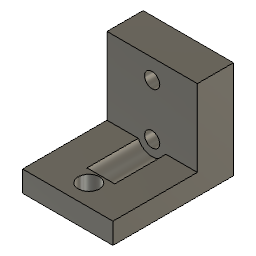
VerbindungMotorisierteLinearfuehrungQuerprofil (Autodesk Fusion 360 design; units mm, degrees)
part number: 2025-11-29-22-10-42-510
Autodesk Fusion 360 part; units mm, degrees
sketch "Skizze1" plane through (0, 0, 0) normal (0, 0, 1) x (1, 0, 0)
  line L0 (0, 0) -> (30, 0)
  line L1 (30, 0) -> (30, 40)
  line L2 (30, 40) -> (0, 40)
  line L3 (0, 40) -> (0, 0)
  dimension "d1" = 30
  dimension "d2" = 40
  constraint horizontal L0
  constraint vertical L1
  constraint horizontal L2
  constraint vertical L3
  constraint coincident L0.start L3.end
  measures "d1" distance of L0.start L0.end
  measures "d2" distance of L0.start L2.end
extrude "Extrusion1" add sketch "Skizze1" along normal blind 7 makes body 1
sketch "Skizze2" plane through (0, 0, 7) normal (0, 0, 1) x (-1, 0, 0)
  line L0 (0, -40) -> (0, 0)
  line L1 (0, 0) -> (-30, 0)
  line L2 (-30, 0) -> (-30, -40)
  line L3 (-30, -40) -> (0, -40)
  line L4 (0, -40) -> (-30, -40)
  line L5 (-30, -40) -> (-30, -28)
  line L6 (-30, -28) -> (0, -28)
  line L7 (0, -28) -> (0, -40)
  constraint horizontal L4
  constraint vertical L5
  constraint horizontal L6
  constraint vertical L7
  constraint coincident L2 L5.end
  constraint coincident L0.start L3.end
extrude "Extrusion2" add sketch "Skizze2" along normal blind 29 contours L0 L2 L3 L4 L5 L6 L7 bodies 1
sketch "Skizze3" plane through (0, 40, 0) normal (0, 1, 0) x (-1, 0, 0)
  line L0 (-30, 0) -> (0, 0)
  line L1 (0, 0) -> (0, 36)
  line L2 (0, 36) -> (-30, 36)
  line L3 (-30, 36) -> (-30, 0)
  line L4 (-15, 0) -> (-15, 36)
  line L5 (-15, 0) -> (-15, 13.5)
  circle A0 centre (-15, 13.5) radius 2.5
  line L6 (-15, 13.5) -> (-15, 30.5)
  circle A1 centre (-15, 30.5) radius 2.5
  dimension "d7" = 13.5
  dimension "d8" = 5
  dimension "d9" = 17
  dimension "d10" = 5
  constraint midpoint L0 L4.start
  constraint midpoint L2 L4.end
  constraint perpendicular L0 L5
  constraint coincident L5.end A0.centre
  constraint parallel L4 L6
  constraint coincident L6.end A1.centre
  measures "d7" distance of L4.start L5.end
  measures "d8" diameter of A0
  measures "d9" distance of L5.end L6.end
  measures "d10" diameter of A1
extrude "Extrusion3" add 1 faces at (20, 32, 36) along direction (0, 0, 1) blind 1 on bodies 1 bodies 1
extrude "Extrusion4" cut sketch "Skizze3" against normal blind 18 contours L4 L5 A0 L6 | L4 L5 A0 L6 | L4 L6 A1 | L4 L6 A1 bodies 1
sketch "Skizze4" plane through (0, 0, 7) normal (0, 0, 1) x (-1, 0, 0)
  line L0 (-30, -28) -> (0, -28)
  line L1 (0, -28) -> (0, 0)
  line L2 (0, 0) -> (-30, 0)
  line L3 (-30, 0) -> (-30, -28)
  line L4 (-15, -28) -> (-15, 0)
  line L5 (-15, 0) -> (-15, -7)
  circle A0 centre (-15, -7) radius 3.5
  line L6 (-15, -7) -> (-15, -21)
  circle A1 centre (-15, -21) radius 3.5
  dimension "d15" = 7
  dimension "d16" = 7
  dimension "d17" = 14
  dimension "d18" = 7
  constraint midpoint L0 L4.start
  constraint midpoint L2 L4.end
  constraint parallel L4 L5
  constraint coincident L5.end A0.centre
  constraint parallel L4 L6
  constraint coincident L6.end A1.centre
  measures "d15" distance of L4.end L5.end
  measures "d16" diameter of A0
  measures "d17" distance of L5.end L6.end
  measures "d18" diameter of A1
extrude "Extrusion5" cut sketch "Skizze4" against normal blind 7 contours L4 L5 A0 L6 | L4 L5 A0 L6 bodies 1
split "Teilen1" by plane through (0, 0, 7) normal (0, 0, 1) bodies 1 makes body 2 at (25.7508, 28, 24.4718)
move_body "Verschieben1" bodies 2 to x (1, 0, 0) y (0, 1, 0) z (0, 0, 1) at (0, 0, -4.5)
sketch "Skizze5" plane through (0, 0, 7) normal (0, 0, 1) x (-1, 0, 0)
  circle A0 centre (-15, -7) radius 3.5
  line L0 (0, -40) -> (0, 0)
  line L1 (0, 0) -> (-30, 0)
  line L2 (-30, 0) -> (-30, -40)
  line L3 (-30, -40) -> (0, -40)
  line L4 (0, -28) -> (-30, -28)
  line L5 (-15, -28) -> (-15, -14)
  constraint coincident L0 L4.start
  constraint coincident L2 L4.end
  constraint perpendicular L2 L4
  constraint midpoint L4 L5.start
  constraint perpendicular L4 L5
sketch "Skizze6" plane through (0, 28, 0) normal (0, -1, 0) x (1, 0, 0)
  circle A0 centre (15, 26) radius 2.5
  circle A1 centre (15, 9) radius 2.5
  line L0 (0, 2.5) -> (30, 2.5)
  line L1 (30, 2.5) -> (30, 32.5)
  line L2 (30, 32.5) -> (0, 32.5)
  line L3 (0, 32.5) -> (0, 2.5)
  circle A2 centre (15, 9) radius 2.5
  circle A3 centre (15, 9) radius 5
  dimension "d23" = 10
  constraint concentric A1 A2
  constraint concentric A1 A3
  measures "d23" diameter of A3
extrude "Extrusion6" cut sketch "Skizze6" along normal blind 14 contours A1 A2 bodies 1
extrude "Extrusion7" cut sketch "Skizze6" along normal blind 14 contours A3 bodies 1
sketch "Skizze7" plane through (0, 40, 0) normal (0, 1, 0) x (-1, 0, 0)
  line L0 (-30, 2.5) -> (0, 2.5)
  line L1 (0, 2.5) -> (0, 32.5)
  line L2 (0, 32.5) -> (-30, 32.5)
  line L3 (-30, 32.5) -> (-30, 2.5)
  circle A0 centre (-15, 26) radius 2.5
  circle A1 centre (-15, 9) radius 2.5
  circle A2 centre (-15, 9) radius 2.5
  constraint concentric A1 A2
extrude "Extrusion8" cut sketch "Skizze6" against normal blind 14.5 contours A1 A2 bodies 1
extrude "Extrusion9" cut 1 faces at (15.2407, 14, 5.2) along direction (0, -1, 0) blind 3 on bodies 1 bodies 1
combine "Kombinieren1" operation add target body 2 tool bodies 1
